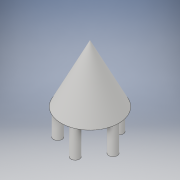
# Autodesk Inventor part: 零件5
Saved by Autodesk Inventor 2019 (Build 230136000, 136)
## iProperties
Created: 2018-12-21
Part Number: 零件5
Material: 一般
Document SubType Name: Modeling
Designer: j13tw
Density: 1 g/cm^3
Appearance: 預設
Author: j13tw
Autodesk Inventor part; units mm, degrees
ref_plane "YZ Plane" through (0, 0, 0) normal (1, 0, 0) x (0, 1, 0)
ref_plane "XZ Plane" through (0, 0, 0) normal (0, 1, 0) x (-1, 0, 0)
ref_plane "XY Plane" through (0, 0, 0) normal (0, 0, 1) x (1, 0, 0)
sketch "草圖1" plane through (0, 0, 0) normal (1, 0, 0) x (0, 1, 0)
  line L0 (12.7, 0) -> (-12.7, -12.7)
  line L1 (12.7, 0) -> (6.35, 0)
  line L2 (-12.7, -5.6796) -> (-12.7, -12.7)
  line L3 (-12.7, -5.6796) -> (6.35, 0)
  line L4 (18.1647, 0) -> (-20.7914, 0)
  point P0 (0, 0)
  dimension "d2" = 12.7
  dimension "d3" = 12.7
  dimension "d5" = 6.35
  dimension "d7" = 12.7
  constraints: 10 end point, 2 horizontal, 1 perpendicular
  measures "d2" distance of point (0, 0) L0.start
  measures "d3" horizontal distance of point (0, 0) L0.end
  measures "d5" distance of L1.end L0.start
  measures "d7" horizontal distance of point (0, 0) L2.start
revolve "迴轉1" add sketch "草圖1" angle 360 about axis through (0, 18.1647, 0) along (0, -1, 0)
sketch "草圖3" plane through (0, -12.7, 0) normal (0, -1, 0) x (1, 0, 0)
  circle A0 centre (10.16, 0) radius 1.905
  circle A1 centre (0, 0) radius 2.7246
  circle A2 centre (3.1396, -9.6627) radius 1.905
  circle A3 centre (0, 0) radius 2.7246
  circle A4 centre (-8.2196, -5.9719) radius 1.905
  circle A5 centre (0, 0) radius 2.7246
  circle A6 centre (-8.2196, 5.9719) radius 1.905
  circle A7 centre (0, 0) radius 2.7246
  circle A8 centre (3.1396, 9.6627) radius 1.905
  circle A9 centre (0, 0) radius 2.7246
  dimension "d9" = 3.81
  dimension "d10" = 10.16
  dimension "d13" = 360
  constraints: 10 centre point, 3 coincident, 18 other
  measures "d9" diameter of A0
  measures "d10" distance of point (0, 0) A0.centre
extrude "擠出1" add sketch "草圖3" along normal blind 12.7 contours A0 | A2 | A4 | A6 | A8
